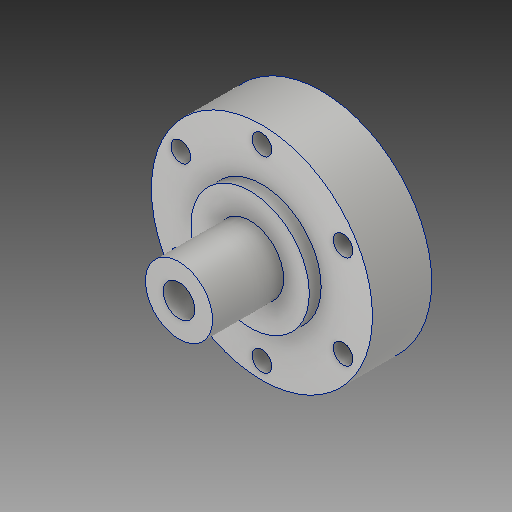
# Autodesk Inventor part: HubOmni1
Saved by Autodesk Inventor 2017 (Build 210142000, 142)
## iProperties
Created: 2020-04-04
Part Number: HubOmni1
Material: Iron, Cast
Document SubType Name: Modeling
Designer: Mochammad Iqbal F
Density: 7.15 g/cm^3
Appearance: Aluminum - Flat
Mass: 297.043 g
Surface Area: 111.495 cm^2
Volume: 41.5444 cm^3
Author: Mochammad Iqbal F
Autodesk Inventor part; units mm, degrees
ref_plane "YZ Plane" through (0, 0, 0) normal (1, 0, 0) x (0, 1, 0)
ref_plane "XZ Plane" through (0, 0, 0) normal (0, 1, 0) x (-1, 0, 0)
ref_plane "XY Plane" through (0, 0, 0) normal (0, 0, 1) x (1, 0, 0)
sketch "Sketch1" plane through (0, 0, 0) normal (0, 0, 1) x (1, 0, 0)
  circle A0 centre (0, 0) radius 28
  line L0 (0, 0) -> (0, 23.75)
  circle A1 centre (0, 23.75) radius 2.5
  circle A2 centre (-20.5681, 11.875) radius 2.5
  circle A3 centre (-20.5681, -11.875) radius 2.5
  circle A4 centre (0, -23.75) radius 2.5
  circle A5 centre (20.5681, -11.875) radius 2.5
  circle A6 centre (20.5681, 11.875) radius 2.5
  dimension "d3" = 56
  dimension "d4" = 23.75
  dimension "d5" = 5
  dimension "d6" = 360
  constraints: 7 centre point, 3 coincident, 2 end point, 1 vertical, 13 other
  measures "d3" diameter of A0
  measures "d4" distance of L0.start L0.end
  measures "d5" diameter of A1
extrude "Extrusion1" add sketch "Sketch1" along normal blind 15
sketch "Sketch2" plane through (0, 0, 15) normal (0, 0, 1) x (1, 0, 0)
  circle A0 centre (0, 0) radius 15
  dimension "d9" = 30
  constraints: 1 centre point, 1 coincident
  measures "d9" diameter of A0
extrude "Extrusion2" add sketch "Sketch2" along normal blind 3
sketch "Sketch3" plane through (0, 0, 18) normal (0, 0, 1) x (1, 0, 0)
  circle A0 centre (0, 0) radius 8.5
  dimension "d12" = 17
  constraints: 1 centre point, 1 coincident
  measures "d12" diameter of A0
extrude "Extrusion3" add sketch "Sketch3" along normal blind 18
sketch "Sketch4" plane through (0, 0, 36) normal (0, 0, 1) x (1, 0, 0)
  circle A0 centre (0, 0) radius 4
  dimension "d15" = 8
  constraints: 1 centre point, 1 coincident
  measures "d15" diameter of A0
extrude "Extrusion4" cut sketch "Sketch4" against normal through all
sketch "Sketch5" plane through (0, 0, 0) normal (0, 0, -1) x (-1, 0, 0)
  circle A0 centre (0, 0) radius 15
  circle A1 centre (0, 0) radius 4 projected
  dimension "d18" = 30
  constraints: 1 centre point, 1 coincident
  measures "d18" diameter of A0
extrude "Extrusion5" add sketch "Sketch5" along normal blind 3
body "Solid1"
